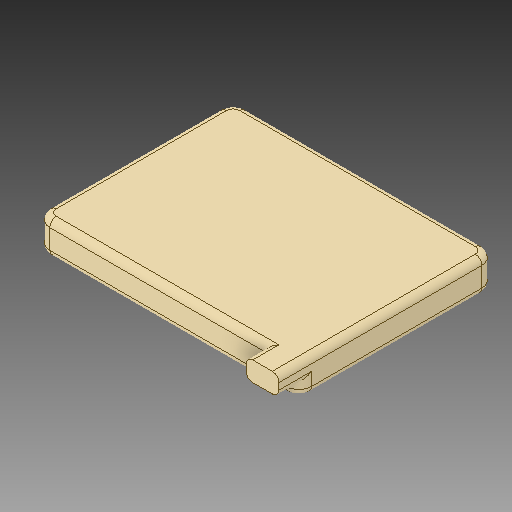
# Autodesk Inventor part: BATTERY_1S_560MAH_AKYGA
Saved by Autodesk Inventor 2018 (Build 220112000, 112)
## iProperties
Created: 2018-08-02
Part Number: BATTERY_1S_560MAH_AKYGA
Material: Generic
Document SubType Name: Modeling
Designer: Luke
Density: 1 g/cm^3
Appearance: Beige
Author: Luke
Autodesk Inventor part; units mm, degrees
ref_plane "YZ Plane" through (0, 0, 0) normal (1, 0, 0) x (0, 1, 0)
ref_plane "XZ Plane" through (0, 0, 0) normal (0, 1, 0) x (-1, 0, 0)
ref_plane "XY Plane" through (0, 0, 0) normal (0, 0, 1) x (1, 0, 0)
sketch "Sketch1" plane through (0, 0, 0) normal (0, 1, 0) x (-1, 0, 0)
  line L0 (0, 0) -> (-40, 0)
  line L1 (-40, 0) -> (-40, -30)
  line L2 (-40, -30) -> (0, -30)
  line L3 (0, -30) -> (0, 0)
  dimension "d0" = 40
  dimension "d1" = 30
  constraints: 8 end point, 2 parallel, 1 horizontal, 1 perpendicular
  measures "d0" distance of L1.end L2.end
  measures "d1" distance of L0.end L1.end
extrude "Extrusion1" add sketch "Sketch1" along normal blind 5
sketch "Sketch2" plane through (0, 0, 0) normal (0, 0, 1) x (1, 0, 0)
  line L0 (0, 0) -> (40, 0) construction
  line L1 (40, 0) -> (40, 5) construction
  line L2 (0, 5) -> (40, 5) construction
  line L3 (0, 0) -> (0, 5) construction
  line L4 (40, 0) -> (40, 5) projected
  line L5 (40, 5) -> (35, 5)
  line L6 (35, 5) -> (35, 2)
  line L7 (35, 2) -> (40, 2)
  line L8 (40, 2) -> (40, 5)
  dimension "d4" = 3
  dimension "d5" = 5
  constraints: 8 end point, 2 parallel, 1 horizontal, 1 perpendicular
  measures "d4" distance of L5.end L6.end
  measures "d5" distance of L6.end L7.end
extrude "Extrusion2" add sketch "Sketch2" along normal blind 3
fillet "Fillet1" radius 2 4 edges at (0, 2.5, 0) (0, 2.5, -30) (40, 2.5, -30) (40, 1, 0)
fillet "Fillet2" radius 1 19 edges at (35, 5, 1.5) (35, 2, 1.5) (40, 2, 1.5) (40, 2, -1) (39.4142, 5, -29.4142) (20, 5, -30) (0.5858, 5, -29.4142) (0, 5, -15) (0.5858, 5, -0.5858) (18.5, 5, 0) (40, 5, -12.5) (40, 0, -15) (39.4142, 0, -29.4142) (20, 0, -30) (0.5858, 0, -29.4142) (0, 0, -15) (0.5858, 0, -0.5858) (20, 0, 0) (39.4142, 0, -0.5858)
body "Solid1"
